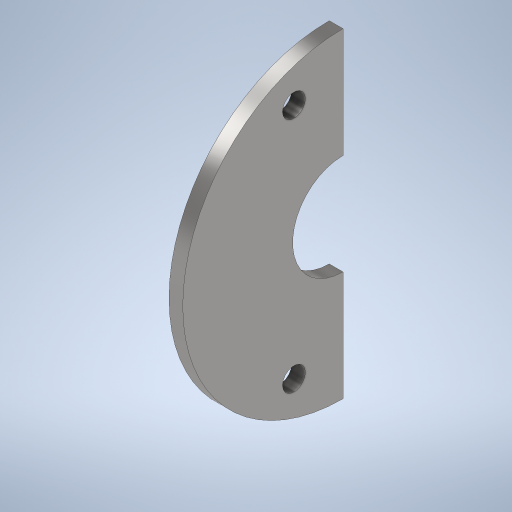
# Autodesk Inventor part: METAL BACKPLATE
Saved by Autodesk Inventor 2023 (Build 270158000, 158)
## iProperties
Created: 2022-09-15
Part Number: METAL BACKPLATE
Material: Steel, Alloy
Document SubType Name: Modeling
Designer: D.C. Eksteen
Density: 7.73 g/cm^3
Appearance: Semi-Polished
Author: D.C. Eksteen
Autodesk Inventor part; units mm, degrees
ref_plane "YZ Plane" through (0, 0, 0) normal (1, 0, 0) x (0, 1, 0)
ref_plane "XZ Plane" through (0, 0, 0) normal (0, 1, 0) x (-1, 0, 0)
ref_plane "XY Plane" through (0, 0, 0) normal (0, 0, 1) x (1, 0, 0)
sketch "Sketch1" plane through (0, 0, 0) normal (1, 0, 0) x (0, 1, 0)
  circle A0 centre (0, 0) radius 35
  dimension "d0" = 70
  constraints: 1 centre point, 1 coincident
  measures "d0" diameter of A0
extrude "Extrusion1" add sketch "Sketch1" along normal blind 3
sketch "Sketch2" plane through (3, 0, 0) normal (1, 0, 0) x (0, 0, -1)
  circle A0 centre (0, 0) radius 11
  circle A1 centre (0, 0) radius 35 projected
  circle A2 centre (0, 0) radius 35 projected
  line L0 (0, 35) -> (0, -35)
  point P0 (0, 11)
  point P1 (0, -11)
  dimension "d3" = 22
  constraints: 2 end point, 2 point on circle, 1 centre point, 1 coincident, 1 midpoint, 1 vertical
  measures "d3" diameter of A0
extrude "Extrusion2" cut sketch "Sketch2" against normal blind 3 contours A0 L0 | A0 L0 A1 | L0 A0 picked at (26.6156, -3.412)
sketch "Sketch3" plane through (3, 0, 0) normal (1, 0, 0) x (0, 0, -1)
  line L0 (0, 11) -> (0, 35) projected
  arc A0 (0, 35) -> (0, -35) centre (0, 0) ccw projected
  line L1 (0, -35) -> (0, -11) projected
  arc A1 (0, 11) -> (0, -11) centre (0, 0) ccw projected
  circle A2 centre (0, 0) radius 28 construction
  line L2 (0, 0) -> (-10.7151, 25.8686)
  line L3 (0, 0) -> (-10.7151, -25.8686)
  dimension "d6" = 56
  dimension "d7" = 22.5
  dimension "d8" = 22.5
  constraints: 4 end point, 3 coincident, 2 point on circle, 1 centre point
  measures "d6" diameter of A2
  measures "d7" angle of L1 L3
  measures "d8" angle of L0 L2
hole "Hole1" at (3, 25.8686, 10.7151) at (3, -25.8686, 10.7151) direction (-1, 0, 0) diameter 5 end through all
body "Solid1"
